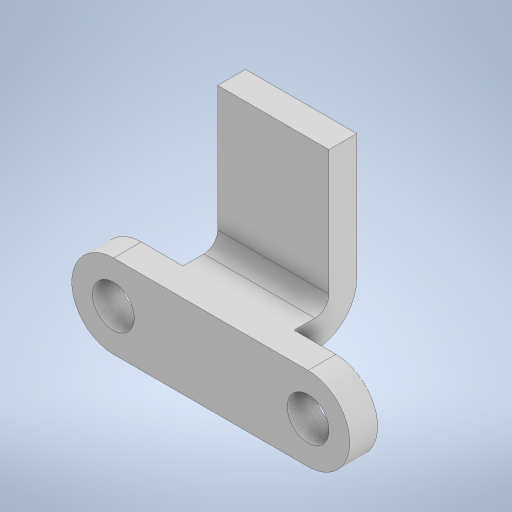
# Autodesk Inventor part: ASN5-6-BK
Saved by Autodesk Inventor 2024 (Build 280153000, 153)
## iProperties
Created: 2023-10-06
Part Number: ASN5-6-BK
Material: Generic
Document SubType Name: Modeling
Designer: bennk
Density: 1 g/cm^3
Appearance: Default
Author: bennk
Autodesk Inventor part; units mm, degrees
ref_plane "YZ Plane" through (0, 0, 0) normal (1, 0, 0) x (0, 1, 0)
ref_plane "XZ Plane" through (0, 0, 0) normal (0, 1, 0) x (-1, 0, 0)
ref_plane "XY Plane" through (0, 0, 0) normal (0, 0, 1) x (1, 0, 0)
sketch "Sketch1" plane through (0, 0, 0) normal (0, 0, 1) x (1, 0, 0)
  line L0 (-88.9, 0) -> (88.9, 0) construction
  line L1 (-88.9, -38.1) -> (88.9, -38.1)
  line L2 (88.9, 38.1) -> (-88.9, 38.1)
  arc A0 (-88.9, 38.1) -> (-88.9, -38.1) centre (-88.9, 0) ccw
  arc A1 (88.9, -38.1) -> (88.9, 38.1) centre (88.9, 0) ccw
  circle A2 centre (-88.9, 0) radius 19.05
  circle A3 centre (88.9, 0) radius 19.05
  point P0 (0, 0)
  point P1 (0, 0)
  dimension "d0" = 177.8
  dimension "d1" = 88.9
  dimension "d2" = 38.1
  dimension "d3" = 38.1
  dimension "d4" = 38.1
  constraints: 8 end point, 4 centre point, 4 point on circle, 4 tangent, 2 coincident, 2 midpoint, 1 horizontal, 1 parallel
  measures "d0" distance of L1.start L1.end
  measures "d1" distance of point (0, 0) L0.end
  measures "d2" radius of A0
  measures "d3" diameter of A2
  measures "d4" diameter of A3
extrude "Extrusion1" add sketch "Sketch1" along normal blind 25.4
sketch "Sketch2" plane through (0, 0, 0) normal (1, 0, 0) x (0, 1, 0)
  line L0 (38.1, 0) -> (-38.1, 0) projected
  line L1 (12.7, 0) -> (38.1, 0)
  line L2 (38.1, 0) -> (38.1, -19.05)
  line L3 (50.8, -31.75) -> (165.1, -31.75)
  line L4 (165.1, -31.75) -> (165.1, -57.15)
  line L5 (165.1, -57.15) -> (50.8, -57.15)
  line L6 (12.7, -19.05) -> (12.7, 0)
  arc A0 (38.1, -19.05) -> (50.8, -31.75) centre (50.8, -19.05) ccw
  arc A1 (12.7, -19.05) -> (50.8, -57.15) centre (50.8, -19.05) ccw
  line L7 (38.1, 0) -> (38.1, 25.4) projected
  line L8 (38.1, 25.4) -> (-38.1, 25.4) projected
  point P0 (0, 0)
  dimension "d7" = 12.7
  dimension "d8" = 38.1
  dimension "d9" = 127
  dimension "d10" = 57.15
  dimension "d11" = 25.4
  dimension "d12" = 25.4
  constraints: 12 end point, 5 perpendicular, 4 point on circle, 4 tangent, 2 centre point, 1 horizontal, 1 point on line
  measures "d7" radius of A0
  measures "d8" radius of A1
  measures "d9" distance between parallel lines of L7 L4
  measures "d10" distance between parallel lines of L8 L3
  measures "d11" distance between parallel lines of L5 L3
  measures "d12" distance between parallel lines of L6 L2
extrude "Extrusion2" add sketch "Sketch2" along normal mid plane 101.6
equation "\"d1\" = 0.5 * d0"
equation "\"d4\" = d3"
body "Solid1"
